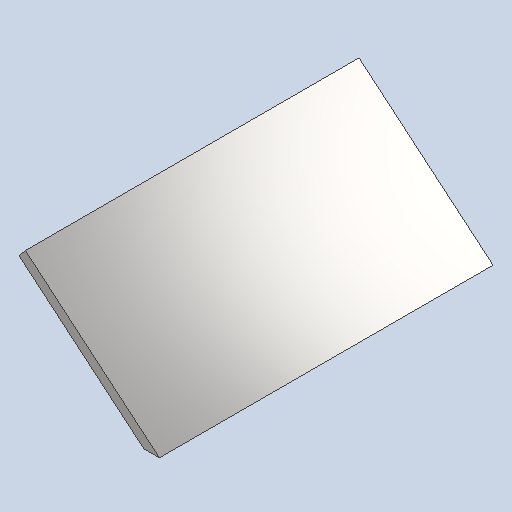
# Autodesk Inventor part: mirror
Saved by Autodesk Inventor 2022 (Build 260153000, 153)
## iProperties
Created: 2022-12-26
Part Number: mirror
Material: Steel, Alloy
Document SubType Name: Modeling
Designer: Kamil
Density: 7.73 g/cm^3
Appearance: Semi-Polished
Author: Kamil
Autodesk Inventor part; units mm, degrees
ref_plane "YZ Plane" through (0, 0, 0) normal (1, 0, 0) x (0, 1, 0)
ref_plane "XZ Plane" through (0, 0, 0) normal (0, 1, 0) x (-1, 0, 0)
ref_plane "XY Plane" through (0, 0, 0) normal (0, 0, 1) x (1, 0, 0)
sketch "Sketch1" plane through (0, 0, 0) normal (0, 0, 1) x (1, 0, 0)
  line L0 (-44.6274, 16.55) -> (3.1619, -23.55) projected
  line L1 (44.6274, -23.55) -> (3.1619, -23.55) projected
  line L2 (44.6274, -23.55) -> (44.6274, -12.55) projected
  line L3 (44.6274, -12.55) -> (28.5274, -12.55) projected
  arc A0 (10.4274, 5.55) -> (28.5274, -12.55) centre (28.5274, 5.55) ccw projected
  line L4 (10.4274, 5.55) -> (10.4274, 16.55) projected
  line L5 (10.4274, 16.55) -> (-44.6274, 16.55) projected
  line L6 (-55.3726, 21.65) -> (-32.3912, 2.3664) projected
  line L7 (-32.3912, 2.3664) -> (-30.4629, 4.6645) projected
  line L8 (-30.4629, 4.6645) -> (-50.7054, 21.65) projected
  line L9 (-50.7054, 21.65) -> (-55.3726, 21.65) projected
  line L10 (-32.3912, 2.3664) -> (12.526, -35.3237)
  line L11 (3.1619, -23.55) -> (14.4544, -33.0256)
  line L12 (14.4544, -33.0256) -> (12.526, -35.3237)
  point P0 (0, 0)
  constraints: 6 end point, 1 perpendicular
ref_plane "Work Plane1" through (-44.6274, -23.55, -100) normal (0, 0, -1) x (0, 1, 0)
extrude "Extrusion1" add sketch "Sketch1" against normal up to surface (100 mm away) contours L0 L11 L12 L10 L7
sketch "Sketch2" plane through (14.4544, -33.0256, -100) normal (0, 0, -1) x (-0.7660444, 0.6427876, 0)
  line L0 (-13.6181, 16.6167) -> (-12.086, 15.3311)
  line L1 (-12.086, 15.3311) -> (12.4819, -5.2838)
  line L2 (0, 0) -> (58.6353, 0) projected
  line L3 (0, -3) -> (0, 0) projected
  line L4 (58.6353, -3) -> (0, -3) projected
  line L5 (58.6353, 0) -> (58.6353, -3) projected
  point P0 (32.3011, 16.0079)
  point P1 (9.7601, -3)
  point P2 (6.1849, 0)
  constraints: 4 end point, 3 other
extrude "Extrusion2" cut sketch "Sketch2" against normal through all contours L1 L4 L3 L2
body "Solid1"
